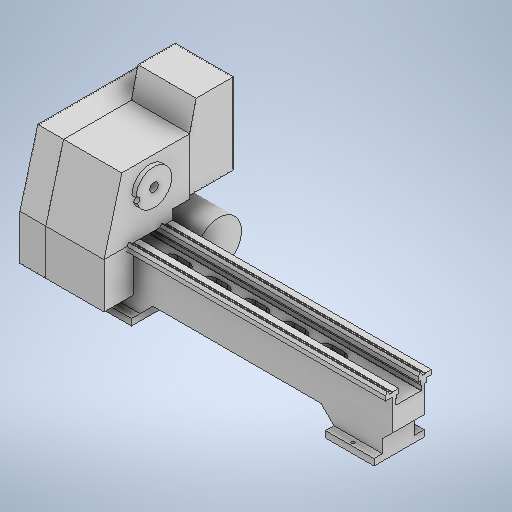
# Autodesk Inventor part: AL-250G Geared Head Lathe
Saved by Autodesk Inventor 2025 (Build 290162010, 162A)
## iProperties
Created: 2024-08-20
Part Number: AL-250G Geared Head Lathe
Material: Generic
Document SubType Name: Modeling
Designer: max_d
Density: 1 g/cm^3
Appearance: Default
Author: max_d
Autodesk Inventor part; units mm, degrees
ref_plane "YZ Plane" through (0, 0, 0) normal (1, 0, 0) x (0, 1, 0)
ref_plane "XZ Plane" through (0, 0, 0) normal (0, 1, 0) x (-1, 0, 0)
sketch "Sketch1" plane through (0, 0, 0) normal (1, 0, 0) x (0, 1, 0)
  line L0 (0, 0) -> (0, 77.5)
  line L1 (0, 77.5) -> (20, 77.5)
  line L2 (20, 77.5) -> (20, 51.5)
  line L3 (20, 51.5) -> (186.35, 51.5)
  line L4 (186.35, 51.5) -> (186.35, 72.1)
  line L5 (186.35, 72.1) -> (200, 72.1)
  line L6 (200, 72.1) -> (208.55, 66.7)
  line L7 (208.55, 66.7) -> (208.55, 64.5)
  line L8 (208.55, 64.5) -> (200, 59.1)
  line L9 (200, 31.5) -> (186, 31.5)
  line L10 (186, 31.5) -> (186, 39)
  line L11 (186, 39) -> (176.5, 39)
  line L12 (159, 39.112) -> (159, -37.762)
  line L13 (0, 0) -> (0, -77.5)
  line L14 (0, -77.5) -> (20, -77.5)
  line L15 (20, -77.5) -> (20, -47.5)
  line L16 (20, -47.5) -> (173, -47.5)
  line L17 (173, -47.5) -> (173, -56)
  line L18 (173, -56) -> (186, -56)
  line L19 (186, -56) -> (186, -69.65)
  line L20 (186, -69.65) -> (200, -69.65)
  line L21 (200, -42.65) -> (208.2, -37.25)
  line L22 (208.2, -37.25) -> (208.2, -35.05)
  line L23 (208.2, -35.05) -> (200, -29.65)
  line L24 (200, -29.65) -> (186, -29.65)
  line L25 (186, -29.65) -> (186, -37.65)
  line L26 (186, -37.65) -> (173.7, -37.65)
  line L27 (200, -42.65) -> (198, -42.65)
  line L28 (198, -42.65) -> (198, -50.65)
  line L29 (198, -50.65) -> (200, -50.65)
  line L30 (200, -50.65) -> (200, -69.65)
  line L31 (200, 59.1) -> (198, 59.1)
  line L32 (198, 59.1) -> (198, 50.8)
  line L33 (198, 50.8) -> (200, 50.8)
  line L34 (200, 50.8) -> (200, 31.5)
  line L35 (200, -42.65) -> (200, -37.25) construction
  line L36 (200, -37.25) -> (208.2, -37.25) construction
  line L37 (200, -29.65) -> (200, -35.05) construction
  line L38 (200, -35.05) -> (208.2, -35.05) construction
  line L39 (200, -35.05) -> (200, -37.25) construction
  line L40 (200, 72.1) -> (200, 66.7) construction
  line L41 (200, 66.7) -> (208.55, 66.7) construction
  line L42 (208.55, 64.5) -> (200, 64.5) construction
  line L43 (200, 64.5) -> (200, 59.1) construction
  line L44 (200, 64.5) -> (200, 66.7) construction
  line L45 (176.5, 39) -> (175.9264, 39.8192)
  line L46 (176.5, 39) -> (177.5, 39) construction
  line L47 (159, 39.112) -> (159.7071, 39.8192)
  line L48 (159, 39.112) -> (160, 39.112) construction
  line L49 (159.7071, 39.8192) -> (175.9264, 39.8192)
  line L50 (159, -37.762) -> (159.7071, -38.4692)
  line L51 (159, -37.762) -> (160, -37.762) construction
  line L52 (159.7071, -38.4692) -> (173.1264, -38.4692)
  line L53 (173.7, -37.65) -> (173.1264, -38.4692)
  line L54 (173.7, -37.65) -> (174.7, -37.65) construction
  dimension "d0" = 155
  dimension "d1" = 20
  dimension "d2" = 20
  dimension "d3" = 26
  dimension "d4" = 30
  dimension "d5" = 153
  dimension "d6" = 8.5
  dimension "d7" = 13.65
  dimension "d8" = 13
  dimension "d9" = 14
  dimension "d10" = 19
  dimension "d11" = 8
  dimension "d12" = 2
  dimension "d13" = 19.3
  dimension "d14" = 14
  dimension "d15" = 7.5
  dimension "d16" = 9.5
  dimension "d17" = 8.3
  dimension "d18" = 2
  dimension "d19" = 20.6
  dimension "d20" = 13.65
  dimension "d21" = 2.2
  dimension "d22" = 2.2
  dimension "d23" = 22.2
  dimension "d24" = 14
  dimension "d25" = 22.2
  dimension "d26" = 13
  dimension "d27" = 13
  dimension "d28" = 12.3
  dimension "d29" = 1
  dimension "d30" = 125
  dimension "d31" = 17.5
  dimension "d32" = 1
  dimension "d33" = 45
  dimension "d34" = 1
  dimension "d35" = 45
  dimension "d36" = 1
  dimension "d37" = 125
  dimension "d38" = 8
  constraints: 110 end point, 27 perpendicular, 8 horizontal, 7 equal length, 5 parallel, 4 point on line, 4 vertical, 3 collinear, 2 vertical alignment
  measures "d0" distance of L13.end L0.end
  measures "d1" distance of L13.end L14.end
  measures "d2" distance of L0.end L1.end
  measures "d3" distance of L1.end L2.end
  measures "d4" distance of L14.end L15.end
  measures "d5" distance of L15.end L16.end
  measures "d6" distance of L16.end L17.end
  measures "d7" distance of L18.end L19.end
  measures "d8" distance of L17.end L18.end
  measures "d9" distance of L19.end L20.end
  measures "d10" distance of L29.end L20.end
  measures "d11" distance of L27.end L28.end
  measures "d12" distance of L28.end L29.end
  measures "d13" distance of L33.end L9.start
  measures "d14" distance of L9.start L9.end
  measures "d15" distance of L9.end L10.end
  measures "d16" distance of L10.end L11.end
  measures "d17" distance of L31.end L32.end
  measures "d18" distance between parallel lines of L34 L32
  measures "d19" distance of L3.end L4.end
  measures "d20" distance of L4.end L5.end
  measures "d21" distance of L6.end L7.end
  measures "d22" distance of L21.end L22.end
  measures "d23" distance between parallel lines of L22 L25
  measures "d24" distance of L23.end L24.end
  measures "d25" distance between parallel lines of L7 L4
  measures "d26" distance between parallel lines of L31 L5
  measures "d27" distance between parallel lines of L27 L24
  measures "d28" distance of L25.end L26.end
  measures "d29" distance of L11.end L45.end
  measures "d30" angle of L46 L45
  measures "d31" distance from line of L12 L11.end
  measures "d32" distance of L12.start L47.end
  measures "d33" angle of L48 L47
  measures "d34" distance of L12.end L50.end
  measures "d35" angle of L50 L51
  measures "d36" distance of L26.end L52.end
  measures "d37" angle of L53 L54
  measures "d38" distance of L24.end L25.end
extrude "Extrusion1" add sketch "Sketch1" against normal blind 980
sketch "Sketch2" plane through (0, 0, 0) normal (0, 0, 1) x (1, 0, 0)
  line L0 (0, 0) -> (-980, 0) construction
  line L1 (0, 0) -> (0, 90) construction
  line L2 (0, 186.35) -> (0, 20) construction
  line L3 (0, 90) -> (-30, 90) construction
  line L4 (-30, 90) -> (-30, 60) construction
  line L5 (0, 90) -> (-30, 60)
  line L6 (-30, 0) -> (0, 0)
  line L7 (0, 0) -> (0, 90)
  line L8 (-30, 60) -> (-30, 0)
  line L9 (-780, 0) -> (-780, 20)
  line L10 (-780, 20) -> (-740, 20) construction
  line L11 (-740, 20) -> (-740, 60) construction
  line L12 (-780, 20) -> (-740, 60)
  line L13 (-30, 0) -> (-180, 0) construction
  line L14 (-180, 0) -> (-180, 20)
  line L15 (-180, 20) -> (-180, 60) construction
  line L16 (-180, 60) -> (-220, 60) construction
  line L17 (-180, 20) -> (-220, 60)
  line L18 (-220, 60) -> (-740, 60)
  line L19 (-780, 0) -> (-180, 0)
  dimension "d42" = 90
  dimension "d43" = 30
  dimension "d44" = 30
  dimension "d48" = 20
  dimension "d49" = 40
  dimension "d50" = 40
  dimension "d51" = 150
  dimension "d52" = 20
  dimension "d53" = 40
  dimension "d54" = 40
  dimension "d59" = 600
  constraints: 36 end point, 6 perpendicular, 5 point on line, 3 vertical, 2 collinear
  measures "d42" distance of L0.start L1.end
  measures "d43" distance of L1.end L3.end
  measures "d44" distance of L3.end L4.end
  measures "d48" distance of L9.start L9.end
  measures "d49" distance of L9.end L10.end
  measures "d50" distance of L10.end L11.end
  measures "d51" distance of L6.start L13.end
  measures "d52" distance of L13.end L14.end
  measures "d53" distance of L14.end L15.end
  measures "d54" distance of L15.end L16.end
  measures "d59" distance of L13.end L9.start
extrude "Extrusion2" cut sketch "Sketch2" along normal mid plane 800
sketch "Sketch3" plane through (-180, 0, 77.5) normal (0, -1, 0) x (1, 0, 0)
  line L0 (-600, -39) -> (0, -39)
  line L1 (0, -39) -> (0, -112)
  line L2 (0, -112) -> (-600, -112)
  line L3 (-600, -112) -> (-600, -39)
  line L4 (-560, -26) -> (-40, -26) projected
  line L5 (-40, -125) -> (-560, -125) projected
  line L6 (0, 0) -> (0, -155) projected
  line L7 (-600, -155) -> (-600, 0) projected
  point P0 (180, -77.5)
  dimension "d55" = 13
  dimension "d56" = 13
  constraints: 8 end point, 2 collinear, 2 parallel, 1 horizontal, 1 perpendicular
  measures "d55" distance between parallel lines of L4 L0
  measures "d56" distance between parallel lines of L5 L2
extrude "Extrusion3" cut sketch "Sketch3" against normal blind 146
sketch "Sketch4" plane through (-180, 146, 77.5) normal (0, -1, 0) x (1, 0, 0)
  line L0 (0, -39) -> (0, -112) construction
  line L1 (0, -75.5) -> (-42.5, -75.5) construction
  line L2 (-42.5, -75.5) -> (-77.5, -75.5) construction
  line L3 (-42.5, -100.5) -> (-77.5, -100.5)
  line L4 (-77.5, -50.5) -> (-42.5, -50.5)
  arc A0 (-42.5, -100.5) -> (-42.5, -50.5) centre (-42.5, -75.5) ccw
  arc A1 (-77.5, -50.5) -> (-77.5, -100.5) centre (-77.5, -75.5) ccw
  line L5 (-197.5, -50.5) -> (-162.5, -50.5)
  arc A2 (-162.5, -100.5) -> (-162.5, -50.5) centre (-162.5, -75.5) ccw
  line L6 (-162.5, -100.5) -> (-197.5, -100.5)
  arc A3 (-197.5, -50.5) -> (-197.5, -100.5) centre (-197.5, -75.5) ccw
  line L7 (-317.5, -50.5) -> (-282.5, -50.5)
  arc A4 (-282.5, -100.5) -> (-282.5, -50.5) centre (-282.5, -75.5) ccw
  line L8 (-282.5, -100.5) -> (-317.5, -100.5)
  arc A5 (-317.5, -50.5) -> (-317.5, -100.5) centre (-317.5, -75.5) ccw
  line L9 (-437.5, -50.5) -> (-402.5, -50.5)
  arc A6 (-402.5, -100.5) -> (-402.5, -50.5) centre (-402.5, -75.5) ccw
  line L10 (-402.5, -100.5) -> (-437.5, -100.5)
  arc A7 (-437.5, -50.5) -> (-437.5, -100.5) centre (-437.5, -75.5) ccw
  line L11 (-557.5, -50.5) -> (-522.5, -50.5)
  arc A8 (-522.5, -100.5) -> (-522.5, -50.5) centre (-522.5, -75.5) ccw
  line L12 (-522.5, -100.5) -> (-557.5, -100.5)
  arc A9 (-557.5, -50.5) -> (-557.5, -100.5) centre (-557.5, -75.5) ccw
  line L13 (-557.5, -75.5) -> (-600, -75.5) construction
  line L14 (-600, -112) -> (-600, -39) construction
  point P0 (180, -77.5)
  point P1 (-60, -75.5)
  dimension "d60" = 35
  dimension "d61" = 50
  dimension "d64" = 120
  constraints: 28 end point, 20 point on circle, 10 centre point, 4 tangent, 3 horizontal, 3 midpoint, 1 collinear, 1 parallel, 40 other
  measures "d60" distance of L1.end L2.end
  measures "d61" distance between parallel lines of L4 L3
  measures "d64" distance of L4.start L5.start
extrude "Extrusion4" cut sketch "Sketch4" against normal blind 36.75
sketch "Sketch5" plane through (-180, 0, 77.5) normal (0, -1, 0) x (1, 0, 0)
  line L0 (150, 0) -> (0, 0) construction
  line L1 (75, 0) -> (75, -155) construction
  line L2 (150, -155) -> (0, -155) construction
  line L3 (-600, 0) -> (-800, 0) construction
  line L4 (-700, 0) -> (-700, -155) construction
  line L5 (-600, -155) -> (-800, -155) construction
  circle A0 centre (75, -10) radius 5
  circle A1 centre (75, -145) radius 5
  circle A2 centre (-700, -10) radius 5
  circle A3 centre (-700, -145) radius 5
  point P0 (180, -77.5)
  dimension "d71" = 10
  dimension "d72" = 10
  dimension "d73" = 10
  dimension "d74" = 10
  dimension "d75" = 10
  constraints: 4 centre point, 4 end point, 4 midpoint, 4 point on line, 3 equal radius
  measures "d71" distance from line of L3 A2.centre
  measures "d72" distance from line of L5 A3.centre
  measures "d73" distance from line of L0 A0.centre
  measures "d74" distance from line of L2 A1.centre
  measures "d75" diameter of A2
extrude "Extrusion5" cut sketch "Sketch5" against normal blind 36.75
ref_plane "Work Plane1" through (-980, 60, -77.5) normal (0, -1, 0) x (1, 0, 0)
sketch "Sketch6" plane through (-980, 60, -77.5) normal (0, -1, 0) x (1, 0, 0)
  line L0 (-80, 220) -> (0, 220)
  line L1 (0, 220) -> (0, -150)
  line L2 (0, -150) -> (-80, -150)
  line L3 (-80, -150) -> (-80, 220)
  line L4 (0, 0) -> (0, 155) projected
  line L5 (200, 0) -> (0, 0) projected
  line L6 (200, 155) -> (0, 155) projected
  point P0 (980, 77.5)
  dimension "d79" = 80
  dimension "d82" = 370
  dimension "d114" = 65
  constraints: 8 end point, 2 parallel, 1 collinear, 1 horizontal, 1 perpendicular
  measures "d79" distance between parallel lines of L3 L4
  measures "d82" distance between parallel lines of L0 L2
  measures "d114" distance between parallel lines of L6 L0
extrude "Extrusion6" add sketch "Sketch6" against normal blind 345 separate body
sketch "Sketch7" plane through (-1060, 60, -227.5) normal (-1, 0, 0) x (0, 0, 1)
  line L0 (370, 345) -> (0, 345) projected
  line L1 (315, 345) -> (370, 140)
  line L2 (370, 0) -> (370, 345) projected
  line L3 (370, 140) -> (370, 345)
  line L4 (370, 345) -> (315, 345)
  point P0 (227.5, -60)
  dimension "d85" = 140
  dimension "d86" = 315
  constraints: 6 end point, 1 collinear, 1 perpendicular, 1 point on line
  measures "d85" distance of L2.start L1.end
  measures "d86" distance of L1.start L0.end
extrude "Extrusion7" cut sketch "Sketch7" against normal up to surface (80 mm away) bodies 2
sketch "Sketch9" plane through (-1060, 60, -227.5) normal (-1, 0, 0) x (0, 0, 1)
  line L0 (0, 345) -> (315, 345) projected
  line L1 (370, 140) -> (315, 345) projected
  line L2 (370, 0) -> (370, 140) projected
  line L3 (370, 0) -> (0, 0) projected
  line L4 (0, 0) -> (0, 345) projected
  line L5 (299.6586, 325) -> (20, 325)
  line L6 (20, 325) -> (20, 20)
  line L7 (20, 20) -> (350, 20)
  line L8 (350, 20) -> (350, 137.3637)
  line L9 (350, 137.3637) -> (299.6586, 325)
  point P0 (227.5, -60)
  dimension "d93" = 20
  constraints: 10 end point, 4 other
  measures "d93" distance between parallel lines of L0 L5
extrude "Extrusion9" cut sketch "Sketch9" against normal blind 78 contours L9 L8 L7 L6 L5 bodies 2
shell "Shell1" thickness 2 removed faces 5 at (-1034, 283.3333, -207.5) at (-1034, 385, -21.061) at (-1008, 259.9091, 105.7195) at (-1034, 119.1212, 122.5) at (-1034, 80, -97.5) bodies 2
sketch "Sketch10" plane through (-1060, 60, -227.5) normal (-1, 0, 0) x (0, 0, 1)
  line L0 (20, 325) -> (299.6586, 325) projected
  line L1 (20, 20) -> (20, 325) projected
  line L2 (299.6586, 325) -> (350, 137.3637) projected
  line L3 (350, 137.3637) -> (350, 20) projected
  line L4 (350, 20) -> (20, 20) projected
  line L5 (301.1927, 327) -> (18, 327)
  line L6 (18, 327) -> (18, 18)
  line L7 (18, 18) -> (352, 18)
  line L8 (352, 18) -> (352, 137.6273)
  line L9 (352, 137.6273) -> (301.1927, 327)
  point P0 (227.5, -60)
  dimension "d97" = 2
  constraints: 10 end point, 4 other
  measures "d97" distance between parallel lines of L0 L5
extrude "Extrusion10" add sketch "Sketch10" against normal blind 15 bodies 2
sketch "Sketch11" plane through (-980, 60, 142.5) normal (1, 0, 0) x (0, 0, -1)
  line L0 (400, 430) -> (400, 180)
  line L1 (400, 180) -> (265, 180)
  line L2 (265, 180) -> (265, 345)
  line L3 (265, 345) -> (285, 430)
  line L4 (285, 430) -> (400, 430)
  line L5 (55, 345) -> (370, 345) projected
  line L6 (370, 0) -> (370, 345) projected
  point P0 (142.5, -60)
  dimension "d100" = 85
  dimension "d101" = 165
  dimension "d102" = 135
  dimension "d103" = 30
  dimension "d104" = 115
  constraints: 10 end point, 2 perpendicular, 1 parallel, 1 point on line, 1 vertical
  measures "d100" distance between parallel lines of L4 L5
  measures "d101" distance between parallel lines of L1 L5
  measures "d102" distance of L0.end L1.end
  measures "d103" distance between parallel lines of L0 L6
  measures "d104" distance of L3.end L0.start
extrude "Extrusion11" add sketch "Sketch11" along normal blind 180 separate body
sketch "Sketch12" plane through (-980, 240, -257.5) normal (0, 0, -1) x (-1, 0, 0)
  line L0 (0, 250) -> (-180, 250) projected
  line L1 (0, 0) -> (0, 250) projected
  line L2 (0, 0) -> (-180, 0) projected
  line L3 (-180, 0) -> (-180, 250) projected
  line L4 (-168, 238) -> (-12, 238)
  line L5 (-12, 238) -> (-12, 12)
  line L6 (-12, 12) -> (-168, 12)
  line L7 (-168, 12) -> (-168, 238)
  point P0 (-980, -240)
  dimension "d107" = 12
  constraints: 8 end point, 3 other
  measures "d107" distance between parallel lines of L0 L4
extrude "Extrusion12" cut sketch "Sketch12" against normal blind 37.25 contours L4 L5 L6 L7 bodies 3
shell "Shell2" thickness 2 removed faces 5 at (-864, 402.6667, -220.25) at (-812, 402.6667, -245.0833) at (-916, 478, -232.6667) at (-968, 327.3333, -245.0833) at (-864, 252, -232.6667) bodies 3
sketch "Sketch13" plane through (-980, 240, -257.5) normal (0, 0, -1) x (-1, 0, 0)
  line L0 (-168, 238) -> (-12, 238) projected
  line L1 (-168, 12) -> (-168, 238) projected
  line L2 (-12, 238) -> (-12, 12) projected
  line L3 (-12, 12) -> (-168, 12) projected
  line L4 (-10, 240) -> (-170, 240)
  line L5 (-170, 240) -> (-170, 10)
  line L6 (-170, 10) -> (-10, 10)
  line L7 (-10, 10) -> (-10, 240)
  point P0 (-980, -240)
  dimension "d111" = 2
  constraints: 8 end point, 3 other
  measures "d111" distance between parallel lines of L0 L4
extrude "Extrusion13" add sketch "Sketch13" against normal blind 12 bodies 3
sketch "Sketch14" plane through (-980, 60, 142.5) normal (1, 0, 0) x (0, 0, -1)
  line L0 (55, 345) -> (0, 140) projected
  line L1 (55, 345) -> (370, 345) projected
  line L2 (265, 345) -> (265, 180) projected
  line L3 (265, 345) -> (265, 170)
  line L4 (265, 170) -> (212.15, 170)
  line L5 (212.15, 140) -> (212.15, 126) projected
  line L6 (212.15, 170) -> (212.15, 140)
  line L7 (265, 180) -> (400, 180) projected
  line L8 (265, 180) -> (265, 345)
  line L9 (55, 345) -> (265, 345)
  line L10 (55, 345) -> (0, 140)
  line L11 (70.4, 140) -> (75.8, 148.55) projected
  line L12 (0, 140) -> (70.4, 140)
  line L13 (70.4, 140) -> (75.8, 148.55)
  line L14 (78, 148.55) -> (83.4, 140) projected
  line L15 (75.8, 148.55) -> (78, 148.55)
  line L16 (78, 148.55) -> (83.4, 140)
  line L17 (91.7, 138) -> (91.7, 140) projected
  line L18 (83.4, 140) -> (91.7, 140)
  line L19 (177.55, 148.2) -> (172.15, 140) projected
  line L20 (91.7, 140) -> (172.15, 140)
  line L21 (172.15, 140) -> (177.55, 148.2)
  line L22 (179.75, 148.2) -> (185.15, 140) projected
  line L23 (177.55, 148.2) -> (179.75, 148.2)
  line L24 (179.75, 148.2) -> (185.15, 140)
  line L25 (193.15, 140) -> (193.15, 138) projected
  line L26 (185.15, 140) -> (193.15, 140)
  line L27 (193.15, 140) -> (212.15, 140)
  point P0 (142.5, -60)
  point P1 (265, 180)
  dimension "d115" = 10
  constraints: 34 end point, 5 collinear, 4 perpendicular, 2 parallel, 2 vertical, 1 horizontal
  measures "d115" distance between parallel lines of L4 L7
extrude "Extrusion14" add sketch "Sketch14" along normal up to surface (180 mm away) separate body
sketch "Sketch15" plane through (-1060, 60, 142.5) normal (0, 0, 1) x (1, 0, 0)
  line L0 (1060, 140) -> (80, 140) projected
  line L1 (80, 140) -> (260, 140)
  line L2 (260, 140) -> (260, 0)
  line L3 (260, 0) -> (80, 0)
  line L4 (80, 0) -> (80, 140)
  line L5 (260, 140) -> (260, 345) projected
  line L6 (80, 0) -> (0, 0) projected
  point P0 (1060, -60)
  constraints: 8 end point, 2 collinear, 2 parallel, 1 horizontal, 1 perpendicular
extrude "Extrusion15" add sketch "Sketch15" against normal up to surface (91 mm away) separate body
sketch "Sketch16" plane through (-980, 60, 142.5) normal (1, 0, 0) x (0, 0, -1)
  circle A0 centre (305, 55) radius 70
  line L0 (190, 30) -> (190, 113) projected
  line L1 (265, 180) -> (400, 180) projected
  point P0 (142.5, -60)
  dimension "d120" = 140
  dimension "d123" = 115
  dimension "d124" = 125
  constraints: 1 centre point
  measures "d120" diameter of A0
  measures "d123" distance from line of A0.centre L0
  measures "d124" distance from line of L1 A0.centre
extrude "Extrusion16" add sketch "Sketch16" along normal blind 230 separate body
sketch "Sketch8" plane through (-980, 60, 142.5) normal (1, 0, 0) x (0, 0, -1)
  circle A0 centre (141.275, 270) radius 13
  line L0 (160.8, 148.55) -> (155.4, 140) construction
  line L1 (212.15, 140) -> (193.15, 140) projected
  line L2 (70.4, 126.35) -> (70.4, 140) construction
  line L3 (70.4, 140) -> (212.15, 140) construction
  line L4 (141.275, 140) -> (141.275, 270) construction
  point P0 (142.5, -60)
  dimension "d90" = 26
  dimension "d126" = 130
  constraints: 4 end point, 1 centre point, 1 midpoint, 1 perpendicular, 1 vertical
  measures "d90" diameter of A0
  measures "d126" distance from line of L4.end L1
extrude "Extrusion8" cut sketch "Sketch8" along normal blind 1042.5 from surface at -2 bodies 2 4
sketch "Sketch17" plane through (-800, 230, -122.5) normal (1, 0, 0) x (0, 0, -1)
  circle A0 centre (-123.725, 100) radius 13 projected
  circle A1 centre (-123.725, 100) radius 55
  circle A2 centre (-123.725, 100) radius 25
  point P0 (-122.5, -230)
  dimension "d127" = 110
  dimension "d134" = 50
  constraints: 2 centre point, 2 coincident
  measures "d127" diameter of A1
  measures "d134" diameter of A2
extrude "Extrusion17" add sketch "Sketch17" along normal blind 13 contours A1 | A2 bodies 4
sketch "Sketch19" plane through (-787, 330, 1.225) normal (1, 0, 0) x (0, 0, -1)
  circle A0 centre (0, 0) radius 55 projected
  circle A1 centre (-54.0833, -10) radius 10
  line L0 (0, 0) -> (-55, 0) construction
  point P0 (1.225, -330)
  point P1 (-55, -0.0421)
  point P2 (-51.3787, -19.6273)
  dimension "d136" = 20
  constraints: 2 end point, 2 point on circle, 1 centre point, 1 horizontal, 1 tangent
  measures "d136" diameter of A1
extrude "Extrusion20" cut sketch "Sketch19" against normal up to surface (13 mm away) contours A1 A0 picked at (-50.7771, -9.2034) bodies 4
sketch "Sketch18" plane through (-774, 330, 1.225) normal (1, 0, 0) x (0, 0, -1)
  circle A0 centre (0, 0) radius 62.5
  circle A1 centre (0, 0) radius 13 projected
  point P0 (1.225, -330)
  dimension "d135" = 125
  constraints: 1 centre point
  measures "d135" diameter of A0
